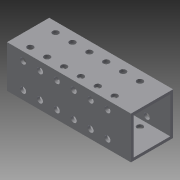
# Autodesk Inventor part: BatHoldV2
Saved by Autodesk Inventor 2015 (Build 190159000, 159)
## iProperties
Created: 2016-03-06
Part Number: BatHoldV2
Material: Generic
Document SubType Name: Modeling
Designer: Hatch
Density: 1 g/cm^3
Appearance: Default
Author: Hatch
Autodesk Inventor part; units mm, degrees
ref_plane "YZ Plane" through (0, 0, 0) normal (1, 0, 0) x (0, 1, 0)
ref_plane "XZ Plane" through (0, 0, 0) normal (0, 1, 0) x (-1, 0, 0)
ref_plane "XY Plane" through (0, 0, 0) normal (0, 0, 1) x (1, 0, 0)
sketch "Sketch1" plane through (0, 0, 0) normal (0, 1, 0) x (-1, 0, 0)
  line L0 (0, 0) -> (88.25, 0)
  line L1 (88.25, 0) -> (88.25, -30)
  line L2 (88.25, -30) -> (0, -30)
  line L3 (0, -30) -> (0, 0)
  dimension "d0" = 88.25
  dimension "d1" = 30
  constraints: 8 end point, 2 parallel, 1 horizontal, 1 perpendicular
  measures "d0" distance of L1.end L2.end
  measures "d1" distance of L0.end L1.end
extrude "Extrusion1" add sketch "Sketch1" along normal blind 2
sketch "Sketch2" plane through (0, 2, 0) normal (0, 1, 0) x (1, 0, 0)
  line L0 (-11.2333, 0) -> (-11.2333, 30)
  line L1 (0, 30) -> (-88.25, 30) projected
  line L2 (-16.7102, 0) -> (-16.7102, 3)
  line L3 (-16.7102, 30) -> (-16.7102, 27)
  line L4 (-16.7102, 3) -> (-16.7102, 5.125)
  circle A0 centre (-16.7102, 5.125) radius 2.125
  line L5 (-16.7102, 15) -> (-76.7102, 15)
  line L6 (-76.7102, 27) -> (-84.8352, 27)
  line L7 (-16.7102, 22.536) -> (-8.5852, 22.536)
  line L8 (-84.8352, 30) -> (-88.25, 30)
  line L9 (-88.25, 30) -> (-88.25, 0)
  line L10 (-88.25, 0) -> (-84.8352, 0)
  line L11 (-84.8352, 0) -> (-84.8352, 30)
  line L12 (-8.5852, 0) -> (0, 0)
  line L13 (0, 0) -> (0, 30)
  line L14 (0, 30) -> (-8.5852, 30)
  line L15 (-8.5852, 30) -> (-8.5852, 0)
  dimension "d4" = 3
  dimension "d5" = 3
  dimension "d6" = 30
  dimension "d7" = 2.125
  dimension "d8" = 4.25
  dimension "d9" = 60
  dimension "d12" = 8.125
  dimension "d13" = 8.125
  constraints: 30 end point, 4 horizontal, 4 parallel, 4 vertical, 3 perpendicular, 3 point on line, 1 centre point, 1 coincident
  measures "d4" distance of L2.start L2.end
  measures "d5" distance of L3.start L3.end
  measures "d6" distance of L0.start L0.end
  measures "d7" distance of L2.end L4.end
  measures "d8" diameter of A0
  measures "d9" distance of L5.start L5.end
  measures "d12" distance of L7.start L7.end
  measures "d13" distance of L6.start L6.end
extrude "Extrusion2" cut sketch "Sketch2" against normal through all contours A0
pattern_linear "Rectangular Pattern1" count 6 spacing 12 along (-1, 0, 0) count 2 spacing 18 along (0, 0, -1) of "Extrusion2"
sketch "Sketch3" plane through (0, 2, 0) normal (0, 1, 0) x (1, 0, 0)
  line L0 (0, 30) -> (0, 0) projected
  line L1 (-88.25, 0) -> (0, 0)
  line L2 (0, 0) -> (0, 2)
  line L3 (0, 2) -> (-88.25, 2)
  line L4 (-88.25, 2) -> (-88.25, 0)
  line L5 (0, 0) -> (0, 30) projected
  line L6 (-88.25, 30) -> (0, 30)
  line L7 (0, 30) -> (0, 28)
  line L8 (0, 28) -> (-88.25, 28)
  line L9 (-88.25, 28) -> (-88.25, 30)
  dimension "d22" = 2
  dimension "d23" = 2
  constraints: 16 end point, 4 parallel, 2 horizontal, 2 perpendicular, 2 point on line
  measures "d22" distance of L2.end L1.end
  measures "d23" distance of L6.end L7.end
extrude "Extrusion3" add sketch "Sketch3" along normal blind 26
sketch "Sketch4" plane through (-88.25, 0, 0) normal (0, 0, 1) x (1, 0, 0)
  line L0 (88.25, 28) -> (0.1331, 28)
  line L1 (0.1331, 28) -> (0.1331, 30)
  line L2 (0.1331, 30) -> (88.25, 30)
  line L3 (88.25, 30) -> (88.25, 28)
  point P0 (88.25, 0)
  dimension "d26" = 2
  constraints: 8 end point, 2 parallel, 1 horizontal, 1 perpendicular
  measures "d26" distance of L0.end L1.end
extrude "Extrusion4" add sketch "Sketch4" against normal blind 30
sketch "Sketch5" plane through (-88.1169, 30, 0) normal (0, 1, 0) x (1, 0, 0)
  circle A0 centre (71.4066, 5.125) radius 2.125 projected
  circle A1 centre (71.4066, 5.125) radius 2.125
  point P0 (88.1169, 0)
  constraints: 1 centre point, 1 coincident
extrude "Extrusion5" cut sketch "Sketch5" against normal through all
pattern_linear "Rectangular Pattern2" count 6 spacing 12 along (-1, 0, 0) count 2 spacing 18 along (0, 0, -1) of "Extrusion5"
sketch "Sketch6" plane through (0, 0, -30) normal (0, 0, -1) x (-1, 0, 0)
  line L0 (18.8352, 0) -> (14.5852, 0) projected
  circle A0 centre (16.7102, 6.1249) radius 2.125
  point P0 (0, 0)
  dimension "d37" = 4.25
  constraints: 1 centre point
  measures "d37" diameter of A0
extrude "Extrusion6" cut sketch "Sketch6" against normal through all
pattern_linear "Rectangular Pattern3" count 6 spacing 12 along (-1, 0, 0) count 2 spacing 18 along (0, 1, 0) of "Extrusion6"
equation "\"d38\" = d37"
body "Solid1"
